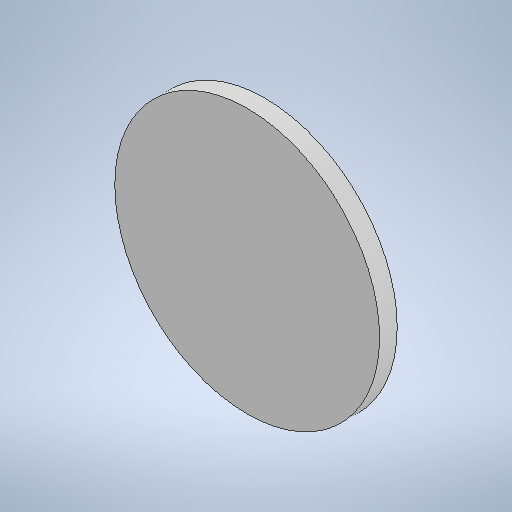
# Autodesk Inventor part: Заглушка фланца трубы подключения фильтра D1000
Saved by Autodesk Inventor 2025 (Build 290162010, 162A)
## iProperties
Created: 2025-02-13
Part Number: Заглушка фланца трубы подключения фильтра D1000
Material: Generic
Document SubType Name: Sheet Metal
Designer: pokla
Density: 1 g/cm^3
Flat Pattern Width: 18 cm
Flat Pattern Length: 18 cm
Flat Pattern Area: 324 cm^2
Sheet Metal Rule: Default
Sheet Metal Width: 180,000 mm
Sheet Metal Length: 180,000 mm
Sheet Metal Area: 32400,000 mm^2
Appearance: Default
Author: pokla
Autodesk Inventor part; units mm, degrees
ref_plane "YZ Plane" through (0, 0, 0) normal (1, 0, 0) x (0, 1, 0)
ref_plane "XZ Plane" through (0, 0, 0) normal (0, 1, 0) x (-1, 0, 0)
ref_plane "XY Plane" through (0, 0, 0) normal (0, 0, 1) x (1, 0, 0)
sketch "Sketch1" plane through (0, 0, 0) normal (0, 1, 0) x (-1, 0, 0)
  circle A0 centre (0, 0) radius 90
  dimension "d4" = 180
  constraints: 1 centre point, 1 coincident
  measures "d4" diameter of A0
extrude "Extrusion1" add sketch "Sketch1" along normal blind 12
equation "\"d4\" = Внешний_диаметр_фланца_трубы_подкл"
equation "\"BendRadius\" = Thickness"
equation "\"BendReliefWidth\" = Thickness"
equation "\"BendReliefDepth\" = 0.5 * Thickness"
equation "\"CornerReliefSize\" = 4 * Thickness"
equation "\"MinimumRemnant\" = 2 * Thickness"
equation "\"TransitionRadius\" = BendRadius"
equation "\"JacobiRadiusSize\" = BendRadius"
equation "\"GapSize\" = Thickness"
equation "\"Внешний_диаметр_фланца_трубы_подкл\" = 180"
equation "\"Thickness\" = 3.048"
body "Solid1"
